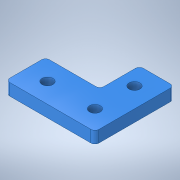
# Autodesk Inventor part: Buffer_Mount
Saved by Autodesk Inventor 2021 (Build 250183000, 183)
## iProperties
Created: 2021-02-02
Part Number: Buffer_Mount
Material: Generic
Document SubType Name: Modeling
Designer: Jorian Brusind
Density: 1 g/cm^3
Appearance: Cyan
Author: Jorian Brusind
Autodesk Inventor part; units mm, degrees
ref_plane "YZ Plane" through (0, 0, 0) normal (1, 0, 0) x (0, 1, 0)
ref_plane "XZ Plane" through (0, 0, 0) normal (0, 1, 0) x (-1, 0, 0)
ref_plane "XY Plane" through (0, 0, 0) normal (0, 0, 1) x (1, 0, 0)
sketch "Sketch1" plane through (0, 0, 0) normal (0, 1, 0) x (-1, 0, 0)
  line L0 (0, 0) -> (45, 0)
  line L1 (45, 0) -> (45, -40)
  line L2 (45, -40) -> (0, -40)
  line L3 (0, -40) -> (0, 0)
  line L4 (45, 0) -> (45, -20)
  line L5 (45, -20) -> (17.5, -20)
  line L6 (17.5, -20) -> (17.5, -40)
  dimension "d0" = 45
  dimension "d1" = 40
  dimension "d13" = 20
  dimension "d14" = 27.5
  constraints: 14 end point, 3 perpendicular, 2 parallel, 1 horizontal, 1 midpoint, 1 point on line
  measures "d0" distance of L1.end L2.end
  measures "d1" distance of L0.end L1.end
  measures "d13" distance of L0.end L4.end
  measures "d14" distance of L4.end L5.end
extrude "Extrusion3" add sketch "Sketch1" along normal blind 6 contours L0 L1 L5 L6 L2 L3
sketch "Sketch5" plane through (0, 6, 0) normal (0, 1, 0) x (1, 0, 0)
  circle A0 centre (-10, 10) radius 2.5
  circle A1 centre (-10, 30) radius 2.5
  line L0 (-45, 0) -> (0, 0) projected
  line L1 (0, 0) -> (0, 40) projected
  dimension "d29" = 5
  dimension "d30" = 5
  dimension "d31" = 10
  dimension "d32" = 10
  dimension "d33" = 10
  dimension "d34" = 20
  constraints: 2 centre point
  measures "d29" diameter of A0
  measures "d30" diameter of A1
  measures "d31" distance from line of L0 A0.centre
  measures "d32" distance from line of L1 A0.centre
  measures "d33" distance from line of L1 A1.centre
  measures "d34" distance of A0.centre A1.centre
extrude "Extrusion5" cut sketch "Sketch5" against normal up to next
sketch "Sketch8" plane through (0, 6, 0) normal (0, 1, 0) x (1, 0, 0)
  circle A0 centre (-10, 10) radius 2.5 projected
  circle A1 centre (-10, 10) radius 2.75
  circle A2 centre (-10, 30) radius 2.5 projected
  circle A3 centre (-10, 30) radius 2.75
  circle A4 centre (-34, 10) radius 2.75
  line L0 (-17.5, 20) -> (-45, 20) projected
  point P0 (0, 0)
  dimension "d42" = 5.5
  dimension "d43" = 5.5
  dimension "d51" = 5.5
  dimension "d52" = 24
  dimension "d53" = 10
  constraints: 3 centre point, 2 coincident
  measures "d42" diameter of A1
  measures "d43" diameter of A3
  measures "d51" diameter of A4
  measures "d52" distance of A1.centre A4.centre
  measures "d53" distance from line of L0 A4.centre
extrude "Extrusion7" cut sketch "Sketch8" against normal blind 10
fillet "Fillet2" radius 2 5 edges at (0, 3, 0) (0, 3, -40) (-17.5, 3, -40) (-17.5, 3, -20) (-17.5, 0, -30)
fillet "Fillet3" radius 2 2 edges at (-45, 3, -20) (-45, 3, 0)
body "Solid2"
